Autodesk Inventor part; units mm, degrees
(part 2 of 2)
  spline S24 degree 3 poles (-22.161672, 44.941631) (-22.171925, 44.941805) (-22.192142, 44.942146) (-22.222099, 44.94568) (-22.251175, 44.951361) (-22.279514, 44.959316) (-22.307263, 44.969053) (-22.334041, 44.981738) (-22.360148, 44.996348) (-22.385514, 45.012986) (-22.409661, 45.032049) (-22.432726, 45.053133) (-22.45413, 45.076764) (-22.474051, 45.10257) (-22.492984, 45.130314) (-22.5104, 45.160373) (-22.526509, 45.192628) (-22.541234, 45.227289) (-22.554289, 45.264861) (-22.565821, 45.305774) (-22.574927, 45.350388) (-22.58272, 45.398346) (-22.589006, 45.449854) (-22.593298, 45.504939) (-22.595951, 45.563567) (-22.596186, 45.603781) (-22.596308, 45.624444) knots 0 0 0 0 0.03378715 0.06662166 0.09928488 0.13136117 0.16358519 0.19610393 0.22890225 0.26215806 0.29599122 0.33021785 0.36505983 0.40095074 0.43762038 0.47570753 0.51538069 0.55641354 0.59976483 0.64642416 0.69643144 0.74978152 0.80657331 0.86743553 0.93188675 1 1 1 1
  spline S25 degree 3 poles (-22.596308, 45.624444) (-22.596186, 45.64528) (-22.595949, 45.685755) (-22.593316, 45.744732) (-22.588943, 45.80006) (-22.582949, 45.851742) (-22.575655, 45.89979) (-22.565917, 45.944077) (-22.554844, 45.984808) (-22.54201, 46.022115) (-22.527529, 46.056501) (-22.511768, 46.088602) (-22.494101, 46.118369) (-22.475538, 46.146277) (-22.455328, 46.17187) (-22.434045, 46.195509) (-22.41086, 46.216647) (-22.38656, 46.235904) (-22.360926, 46.252786) (-22.334687, 46.267655) (-22.307663, 46.280358) (-22.279782, 46.290346) (-22.251292, 46.298595) (-22.222095, 46.304237) (-22.192143, 46.307787) (-22.171925, 46.308126) (-22.161672, 46.308298) knots 0 0 0 0 0.06859462 0.13324604 0.19431259 0.25127922 0.30451344 0.35423491 0.40048059 0.44341075 0.48401487 0.5232523 0.56104237 0.59790024 0.63351849 0.66831435 0.70249567 0.73668535 0.77029317 0.80343726 0.83591295 0.86846025 0.90084654 0.93346652 0.96625758 1 1 1 1
  spline S26 degree 3 poles (-22.161672, 46.308298) (-22.151333, 46.308117) (-22.130772, 46.307757) (-22.100375, 46.304293) (-22.070679, 46.298547) (-22.041812, 46.290405) (-22.013537, 46.280304) (-21.986075, 46.267643) (-21.959255, 46.252905) (-21.933504, 46.235587) (-21.908539, 46.21628) (-21.884972, 46.194454) (-21.862803, 46.170329) (-21.841752, 46.144165) (-21.822417, 46.115459) (-21.804004, 46.084711) (-21.787523, 46.051382) (-21.77165, 46.01603) (-21.757949, 45.977675) (-21.745593, 45.936533) (-21.73561, 45.89212) (-21.727294, 45.844668) (-21.720851, 45.794002) (-21.716159, 45.740232) (-21.713681, 45.683321) (-21.713214, 45.644411) (-21.712974, 45.624444) knots 0 0 0 0 0.03378812 0.06719393 0.09986241 0.13256661 0.16515117 0.19791319 0.231319 0.26508328 0.29925531 0.33439857 0.36994282 0.40628356 0.44406382 0.48299771 0.52335445 0.56553659 0.60961292 0.65639081 0.70588549 0.7583245 0.81383178 0.87279456 0.93472223 1 1 1 1
  line L64 (-27.862974, 45.624965) -> (-27.729641, 46.274965)
  line L65 (-27.729641, 46.274965) -> (-27.196308, 46.274965)
  line L66 (-27.196308, 46.274965) -> (-27.196308, 46.141631)
  line L67 (-27.196308, 46.141631) -> (-27.638495, 46.141631)
  line L68 (-27.638495, 46.141631) -> (-27.708547, 45.799704)
  spline S27 degree 3 poles (-27.708547, 45.799704) (-27.694784, 45.803504) (-27.668119, 45.810866) (-27.628762, 45.819039) (-27.591399, 45.823966) (-27.567154, 45.824639) (-27.555422, 45.824965) knots 0 0 0 0 0.27506837 0.53290146 0.77397346 1 1 1 1
  spline S28 degree 3 poles (-27.555422, 45.824965) (-27.540905, 45.824651) (-27.512362, 45.824033) (-27.470599, 45.8181) (-27.430732, 45.808763) (-27.392846, 45.795718) (-27.356869, 45.779037) (-27.323133, 45.7582) (-27.291131, 45.733859) (-27.261438, 45.705874) (-27.234501, 45.675074) (-27.210816, 45.641959) (-27.190699, 45.606848) (-27.174519, 45.569408) (-27.161599, 45.530052) (-27.153, 45.488365) (-27.147274, 45.444742) (-27.146634, 45.414914) (-27.146308, 45.399704) knots 0 0 0 0 0.06580765 0.12939427 0.19089406 0.25128107 0.31081496 0.37037099 0.43076826 0.49288125 0.55510395 0.61606705 0.67725603 0.73825981 0.80076213 0.86477758 0.93104529 1 1 1 1
  spline S29 degree 3 poles (-27.146308, 45.399704) (-27.146555, 45.38911) (-27.147045, 45.368066) (-27.149541, 45.336812) (-27.154346, 45.30622) (-27.160796, 45.276286) (-27.169169, 45.247066) (-27.179305, 45.218476) (-27.191709, 45.190695) (-27.205315, 45.16346) (-27.220636, 45.137387) (-27.237639, 45.113003) (-27.255603, 45.089943) (-27.274933, 45.068454) (-27.295808, 45.048678) (-27.317974, 45.030498) (-27.341257, 45.013604) (-27.366014, 44.998685) (-27.391696, 44.984956) (-27.418672, 44.973693) (-27.446329, 44.963623) (-27.475064, 44.955597) (-27.504813, 44.949307) (-27.535625, 44.945036) (-27.567338, 44.941925) (-27.588834, 44.94173) (-27.599693, 44.941631) knots 0 0 0 0 0.04401447 0.08743412 0.1301184 0.17255369 0.21455476 0.25629809 0.29843823 0.340849 0.38271519 0.42392405 0.46424624 0.50407367 0.54386191 0.58356672 0.62309432 0.66322906 0.70355126 0.74393789 0.78454125 0.82575011 0.86775736 0.91074516 0.95491445 1 1 1 1
  spline S30 degree 3 poles (-27.599693, 44.941631) (-27.612646, 44.941888) (-27.63813, 44.942393) (-27.675467, 44.947674) (-27.711389, 44.955238) (-27.745609, 44.966617) (-27.778432, 44.980875) (-27.809418, 44.998895) (-27.839357, 45.019316) (-27.867033, 45.043415) (-27.89272, 45.069755) (-27.915714, 45.098339) (-27.936192, 45.128696) (-27.953826, 45.160972) (-27.968869, 45.195084) (-27.980686, 45.231158) (-27.990223, 45.269006) (-27.994258, 45.295063) (-27.996308, 45.308298) knots 0 0 0 0 0.06542114 0.12870837 0.19023614 0.2507244 0.31063718 0.37076641 0.43161474 0.49352297 0.55588346 0.61734237 0.67866804 0.74071136 0.80298536 0.86680258 0.93234717 1 1 1 1
  line L69 (-27.996308, 45.308298) -> (-27.879641, 45.308298)
  spline S31 degree 3 poles (-27.879641, 45.308298) (-27.87677, 45.295901) (-27.871253, 45.272073) (-27.859142, 45.238596) (-27.844335, 45.208763) (-27.826728, 45.18218) (-27.805723, 45.159) (-27.781755, 45.138342) (-27.754883, 45.119706) (-27.725023, 45.104171) (-27.693521, 45.090923) (-27.66055, 45.082101) (-27.627008, 45.075898) (-27.604322, 45.075277) (-27.592922, 45.074965) knots 0 0 0 0 0.09468725 0.18199416 0.26437695 0.34217986 0.41861761 0.49650908 0.57736909 0.66151059 0.74673255 0.83125798 0.91520562 1 1 1 1
  spline S32 degree 3 poles (-27.592922, 45.074965) (-27.581795, 45.07527) (-27.559885, 45.07587) (-27.527641, 45.08049) (-27.49651, 45.087606) (-27.4668, 45.098255) (-27.437992, 45.111197) (-27.410813, 45.127805) (-27.384478, 45.146919) (-27.359804, 45.168817) (-27.337207, 45.192949) (-27.31724, 45.218755) (-27.300609, 45.246284) (-27.286593, 45.27506) (-27.275951, 45.305397) (-27.268358, 45.337155) (-27.2639, 45.370411) (-27.263287, 45.393094) (-27.262974, 45.404652) knots 0 0 0 0 0.0642073 0.12642469 0.18768028 0.24821642 0.30830506 0.36966099 0.43169855 0.49594689 0.55975802 0.62229541 0.68391064 0.74509241 0.80674023 0.86908662 0.93329 1 1 1 1
  spline S33 degree 3 poles (-27.262974, 45.404652) (-27.263219, 45.41508) (-27.263698, 45.435492) (-27.267609, 45.465355) (-27.274412, 45.49361) (-27.283856, 45.520396) (-27.295845, 45.545736) (-27.310497, 45.569657) (-27.328085, 45.591844) (-27.348176, 45.612307) (-27.370186, 45.631192) (-27.394494, 45.647291) (-27.420591, 45.660835) (-27.448162, 45.672523) (-27.477863, 45.680918) (-27.509106, 45.68722) (-27.542229, 45.690866) (-27.564875, 45.691371) (-27.576516, 45.691631) knots 0 0 0 0 0.06535138 0.12791603 0.18836021 0.24721608 0.30563013 0.36376984 0.42266091 0.48268729 0.54330022 0.60411796 0.66496489 0.72741349 0.79146763 0.85805544 0.92703681 1 1 1 1
  spline S34 degree 3 poles (-27.576516, 45.691631) (-27.586592, 45.691416) (-27.607398, 45.690971) (-27.639312, 45.687692) (-27.672849, 45.682403) (-27.70788, 45.675128) (-27.74451, 45.665608) (-27.782663, 45.6542) (-27.822418, 45.64056) (-27.849204, 45.63026) (-27.862974, 45.624965) knots 0 0 0 0 0.10220304 0.21102334 0.32509966 0.4465021 0.57378772 0.70890071 0.85035787 1 1 1 1
  line L70 (0, 0) -> (-7.5, 0)
  circle A17 centre (0, 0) radius 7.5
  line L71 (-11.162974, -50.524965) -> (-11.675559, -50.524965)
  line L72 (-11.675559, -50.524965) -> (-11.767254, -49.090957)
  arc A18 (-11.767254, -49.090957) -> (-15.958694, -49.090957) centre (-13.862974, -49.224965) ccw
  line L73 (-15.958694, -49.090957) -> (-16.05039, -50.524965)
  line L74 (-16.05039, -50.524965) -> (-20.33871, -50.524965)
  arc A19 (-20.409421, -50.495675) -> (-20.33871, -50.524965) centre (-20.33871, -50.424965) ccw
  line L75 (-20.409421, -50.495675) -> (-20.733685, -50.171411)
  arc A20 (-20.733685, -50.171411) -> (-21.087238, -50.024965) centre (-21.087238, -50.524965) ccw
  line L76 (-21.087238, -50.024965) -> (-30.762974, -50.024965)
  arc A21 (-30.862974, -49.924965) -> (-30.762974, -50.024965) centre (-30.762974, -49.924965) ccw
  line L77 (-30.862974, -49.924965) -> (-30.862974, -40.774965)
  arc A22 (-30.762974, -40.674965) -> (-30.862974, -40.774965) centre (-30.762974, -40.774965) ccw
  line L78 (-30.762974, -40.674965) -> (-27.837238, -40.674965)
  arc A23 (-27.837238, -40.674965) -> (-27.483685, -40.528518) centre (-27.837238, -40.174965) ccw
  line L79 (-27.483685, -40.528518) -> (-27.159421, -40.204254)
  arc A24 (-27.08871, -40.174965) -> (-27.159421, -40.204254) centre (-27.08871, -40.274965) ccw
  line L80 (-27.08871, -40.174965) -> (-24.337238, -40.174965)
  arc A25 (-24.266528, -40.204254) -> (-24.337238, -40.174965) centre (-24.337238, -40.274965) ccw
  line L81 (-24.266528, -40.204254) -> (-23.942264, -40.528518)
  arc A26 (-23.942264, -40.528518) -> (-23.58871, -40.674965) centre (-23.58871, -40.174965) ccw
  line L82 (-23.58871, -40.674965) -> (-18.337238, -40.674965)
  arc A27 (-18.337238, -40.674965) -> (-17.983685, -40.528518) centre (-18.337238, -40.174965) ccw
  line L83 (-17.983685, -40.528518) -> (-17.659421, -40.204254)
  arc A28 (-17.58871, -40.174965) -> (-17.659421, -40.204254) centre (-17.58871, -40.274965) ccw
  line L84 (-17.58871, -40.174965) -> (-14.837238, -40.174965)
  arc A29 (-14.766528, -40.204254) -> (-14.837238, -40.174965) centre (-14.837238, -40.274965) ccw
  line L85 (-14.766528, -40.204254) -> (-14.442264, -40.528518)
  arc A30 (-14.442264, -40.528518) -> (-14.08871, -40.674965) centre (-14.08871, -40.174965) ccw
  line L86 (-14.08871, -40.674965) -> (-11.162974, -40.674965)
  arc A31 (-11.062974, -40.774965) -> (-11.162974, -40.674965) centre (-11.162974, -40.774965) ccw
  line L87 (-11.062974, -40.774965) -> (-11.062974, -50.424965)
  arc A32 (-11.162974, -50.524965) -> (-11.062974, -50.424965) centre (-11.162974, -50.424965) ccw
  circle A33 centre (-16.212974, -42.724965) radius 1.25
  circle A34 centre (-25.712974, -42.724965) radius 1.25
  line L88 (-26.886308, -44.974965) -> (-26.269641, -46.274965)
  line L89 (-26.269641, -46.274965) -> (-26.252974, -46.274965)
  line L90 (-26.252974, -46.274965) -> (-25.652974, -44.974965)
  line L91 (-25.652974, -44.974965) -> (-25.779797, -44.974965)
  line L92 (-25.779797, -44.974965) -> (-25.971985, -45.391631)
  line L93 (-25.971985, -45.391631) -> (-26.561308, -45.391631)
  line L94 (-26.561308, -45.391631) -> (-26.758964, -44.974965)
  line L95 (-26.758964, -44.974965) -> (-26.886308, -44.974965)
  spline S35 degree 3 poles (-24.066308, -45.911423) (-24.066544, -45.920293) (-24.067009, -45.937775) (-24.071116, -45.963406) (-24.077323, -45.98813) (-24.086217, -46.012023) (-24.097957, -46.034846) (-24.112247, -46.056625) (-24.128734, -46.077681) (-24.147808, -46.097424) (-24.168761, -46.115506) (-24.190896, -46.131523) (-24.214314, -46.144909) (-24.238918, -46.155882) (-24.264637, -46.16449) (-24.291523, -46.170455) (-24.319501, -46.1742) (-24.338605, -46.174707) (-24.348339, -46.174965) knots 0 0 0 0 0.0619654 0.12212191 0.1809885 0.23993322 0.29990583 0.35998885 0.42177574 0.48657583 0.5515348 0.61501754 0.67725862 0.73972996 0.8030501 0.86649513 0.93197347 1 1 1 1
  spline S36 degree 3 poles (-24.348339, -46.174965) (-24.358505, -46.174699) (-24.37847, -46.174178) (-24.407783, -46.170529) (-24.435746, -46.164235) (-24.46243, -46.155627) (-24.48788, -46.144685) (-24.511973, -46.131056) (-24.534653, -46.114794) (-24.555965, -46.096356) (-24.5756, -46.075828) (-24.592851, -46.052944) (-24.607926, -46.028123) (-24.621078, -46.00143) (-24.631758, -45.972625) (-24.63992, -45.941808) (-24.646378, -45.909114) (-24.648535, -45.886537) (-24.649641, -45.874965) knots 0 0 0 0 0.06443867 0.12654691 0.18688715 0.24587754 0.30404088 0.36219122 0.42097593 0.48066028 0.54060027 0.6006891 0.66193579 0.72444251 0.78903839 0.85631376 0.92635203 1 1 1 1
  line L96 (-24.649641, -45.874965) -> (-24.766308, -45.874965)
  spline S37 degree 3 poles (-24.766308, -45.874965) (-24.765547, -45.890443) (-24.764054, -45.92084) (-24.757061, -45.965161) (-24.747054, -46.007524) (-24.732906, -46.04759) (-24.715335, -46.085713) (-24.694264, -46.121741) (-24.669306, -46.155538) (-24.641001, -46.18679) (-24.610258, -46.215459) (-24.577087, -46.240217) (-24.54223, -46.261135) (-24.505793, -46.278622) (-24.467365, -46.291749) (-24.427294, -46.301488) (-24.385405, -46.307348) (-24.356865, -46.307978) (-24.342349, -46.308298) knots 0 0 0 0 0.06879079 0.13510329 0.19897867 0.2619043 0.32349497 0.38519538 0.44696924 0.50976478 0.57225057 0.63340518 0.69325116 0.75258316 0.81257927 0.87327508 0.93554994 1 1 1 1
  spline S38 degree 3 poles (-24.342349, -46.308298) (-24.328095, -46.307964) (-24.300085, -46.307309) (-24.259204, -46.301677) (-24.220287, -46.292858) (-24.183409, -46.280483) (-24.148864, -46.263849) (-24.116392, -46.243867) (-24.085608, -46.220757) (-24.057897, -46.193548) (-24.032451, -46.164502) (-24.010499, -46.133492) (-23.9917, -46.101464) (-23.97603, -46.068173) (-23.964495, -46.033307) (-23.955737, -45.997372) (-23.950787, -45.959998) (-23.950027, -45.934701) (-23.949641, -45.92184) knots 0 0 0 0 0.06947546 0.1365168 0.20078882 0.26382967 0.32573502 0.38729069 0.44950922 0.51296782 0.57627522 0.6375801 0.69790261 0.75717209 0.81659853 0.87665317 0.93728964 1 1 1 1
  spline S39 degree 3 poles (-23.949641, -45.92184) (-23.95027, -45.903733) (-23.951517, -45.867838) (-23.962182, -45.81509) (-23.978839, -45.763984) (-23.998895, -45.722853) (-24.019128, -45.689709) (-24.037361, -45.662421) (-24.058705, -45.633039) (-24.083471, -45.601661) (-24.111147, -45.568043) (-24.141984, -45.532204) (-24.176201, -45.494514) (-24.200217, -45.468772) (-24.212662, -45.455434) knots 0 0 0 0 0.0987022 0.19567231 0.29242243 0.39134254 0.44446244 0.50422878 0.57035234 0.64254575 0.72228751 0.80792112 0.90046954 1 1 1 1
  line L97 (-24.212662, -45.455434) -> (-24.537922, -45.108298)
  line L98 (-24.537922, -45.108298) -> (-23.932974, -45.108298)
  line L99 (-23.932974, -45.108298) -> (-23.932974, -44.974965)
  line L100 (-23.932974, -44.974965) -> (-24.816308, -44.974965)
  line L101 (-24.816308, -44.974965) -> (-24.312141, -45.512986)
  spline S40 degree 3 poles (-24.312141, -45.512986) (-24.299866, -45.525799) (-24.276288, -45.550412) (-24.242941, -45.586345) (-24.212989, -45.61968) (-24.18624, -45.650355) (-24.163273, -45.678818) (-24.142892, -45.704148) (-24.126562, -45.727457) (-24.108839, -45.754475) (-24.091674, -45.787462) (-24.076923, -45.827775) (-24.067929, -45.869273) (-24.06685, -45.897317) (-24.066308, -45.911423) knots 0 0 0 0 0.11080264 0.2128292 0.30610131 0.39064732 0.46692447 0.53448104 0.59358694 0.644557 0.73620045 0.82502403 0.91198558 1 1 1 1
  line L102 (-23.556308, -45.624965) -> (-23.422974, -46.274965)
  line L103 (-23.422974, -46.274965) -> (-22.889641, -46.274965)
  line L104 (-22.889641, -46.274965) -> (-22.889641, -46.141631)
  line L105 (-22.889641, -46.141631) -> (-23.331828, -46.141631)
  line L106 (-23.331828, -46.141631) -> (-23.401881, -45.799704)
  spline S41 degree 3 poles (-23.401881, -45.799704) (-23.388117, -45.803504) (-23.361452, -45.810866) (-23.322096, -45.819039) (-23.284733, -45.823966) (-23.260488, -45.824639) (-23.248756, -45.824965) knots 0 0 0 0 0.27506837 0.53290146 0.77397346 1 1 1 1
  spline S42 degree 3 poles (-23.248756, -45.824965) (-23.234239, -45.824651) (-23.205695, -45.824033) (-23.163932, -45.8181) (-23.124065, -45.808763) (-23.086179, -45.795718) (-23.050202, -45.779037) (-23.016466, -45.7582) (-22.984465, -45.733859) (-22.954772, -45.705874) (-22.927834, -45.675074) (-22.90415, -45.641959) (-22.884032, -45.606848) (-22.867852, -45.569408) (-22.854932, -45.530052) (-22.846333, -45.488365) (-22.840607, -45.444742) (-22.839967, -45.414914) (-22.839641, -45.399704) knots 0 0 0 0 0.06580765 0.12939427 0.19089406 0.25128107 0.31081496 0.37037099 0.43076826 0.49288125 0.55510395 0.61606705 0.67725603 0.73825981 0.80076213 0.86477758 0.93104529 1 1 1 1
  spline S43 degree 3 poles (-22.839641, -45.399704) (-22.839888, -45.38911) (-22.840379, -45.368066) (-22.842874, -45.336812) (-22.847679, -45.30622) (-22.85413, -45.276286) (-22.862503, -45.247066) (-22.872639, -45.218476) (-22.885043, -45.190695) (-22.898649, -45.16346) (-22.913969, -45.137387) (-22.930972, -45.113003) (-22.948937, -45.089943) (-22.968266, -45.068454) (-22.989141, -45.048678) (-23.011308, -45.030498) (-23.03459, -45.013604) (-23.059348, -44.998685) (-23.085029, -44.984956) (-23.112005, -44.973693) (-23.139662, -44.963623) (-23.168398, -44.955597) (-23.198147, -44.949307) (-23.228959, -44.945036) (-23.260671, -44.941925) (-23.282168, -44.94173) (-23.293026, -44.941631) knots 0 0 0 0 0.04401447 0.08743412 0.1301184 0.17255369 0.21455476 0.25629809 0.29843823 0.340849 0.38271519 0.42392405 0.46424624 0.50407367 0.54386191 0.58356672 0.62309432 0.66322906 0.70355126 0.74393789 0.78454125 0.82575011 0.86775736 0.91074516 0.95491445 1 1 1 1
  spline S44 degree 3 poles (-23.293026, -44.941631) (-23.30598, -44.941888) (-23.331464, -44.942393) (-23.3688, -44.947674) (-23.404722, -44.955238) (-23.438942, -44.966617) (-23.471766, -44.980875) (-23.502751, -44.998895) (-23.532691, -45.019316) (-23.560367, -45.043415) (-23.586053, -45.069755) (-23.609047, -45.098339) (-23.629525, -45.128696) (-23.64716, -45.160972) (-23.662202, -45.195084) (-23.674019, -45.231158) (-23.683557, -45.269006) (-23.687592, -45.295063) (-23.689641, -45.308298) knots 0 0 0 0 0.06542114 0.12870837 0.19023614 0.2507244 0.31063718 0.37076641 0.43161474 0.49352297 0.55588346 0.61734237 0.67866804 0.74071136 0.80298536 0.86680258 0.93234717 1 1 1 1
  line L107 (-23.689641, -45.308298) -> (-23.572974, -45.308298)
  spline S45 degree 3 poles (-23.572974, -45.308298) (-23.570104, -45.295901) (-23.564586, -45.272073) (-23.552475, -45.238596) (-23.537668, -45.208763) (-23.520061, -45.18218) (-23.499057, -45.159) (-23.475088, -45.138342) (-23.448216, -45.119706) (-23.418356, -45.104171) (-23.386854, -45.090923) (-23.353883, -45.082101) (-23.320342, -45.075898) (-23.297656, -45.075277) (-23.286256, -45.074965) knots 0 0 0 0 0.09468725 0.18199416 0.26437695 0.34217986 0.41861761 0.49650908 0.57736909 0.66151059 0.74673255 0.83125798 0.91520562 1 1 1 1
  spline S46 degree 3 poles (-23.286256, -45.074965) (-23.275128, -45.07527) (-23.253218, -45.07587) (-23.220974, -45.08049) (-23.189843, -45.087606) (-23.160134, -45.098255) (-23.131325, -45.111197) (-23.104146, -45.127805) (-23.077811, -45.146919) (-23.053138, -45.168817) (-23.03054, -45.192949) (-23.010574, -45.218755) (-22.993942, -45.246284) (-22.979927, -45.27506) (-22.969284, -45.305397) (-22.961692, -45.337155) (-22.957233, -45.370411) (-22.95662, -45.393094) (-22.956308, -45.404652) knots 0 0 0 0 0.0642073 0.12642469 0.18768028 0.24821642 0.30830506 0.36966099 0.43169855 0.49594689 0.55975802 0.62229541 0.68391064 0.74509241 0.80674023 0.86908662 0.93329 1 1 1 1
  spline S47 degree 3 poles (-22.956308, -45.404652) (-22.956552, -45.41508) (-22.957031, -45.435492) (-22.960942, -45.465355) (-22.967746, -45.49361) (-22.977189, -45.520396) (-22.989178, -45.545736) (-23.00383, -45.569657) (-23.021418, -45.591844) (-23.04151, -45.612307) (-23.06352, -45.631192) (-23.087827, -45.647291) (-23.113924, -45.660835) (-23.141495, -45.672523) (-23.171196, -45.680918) (-23.202439, -45.68722) (-23.235562, -45.690866) (-23.258209, -45.691371) (-23.269849, -45.691631) knots 0 0 0 0 0.06535138 0.12791603 0.18836021 0.24721608 0.30563013 0.36376984 0.42266091 0.48268729 0.54330022 0.60411796 0.66496489 0.72741349 0.79146763 0.85805544 0.92703681 1 1 1 1
  spline S48 degree 3 poles (-23.269849, -45.691631) (-23.279926, -45.691416) (-23.300731, -45.690971) (-23.332645, -45.687692) (-23.366182, -45.682403) (-23.401213, -45.675128) (-23.437844, -45.665608) (-23.475996, -45.6542) (-23.515751, -45.64056) (-23.542538, -45.63026) (-23.556308, -45.624965) knots 0 0 0 0 0.10220304 0.21102334 0.32509966 0.4465021 0.57378772 0.70890071 0.85035787 1 1 1 1
  line L108 (-20.109641, -44.974965) -> (-19.492974, -46.274965)
  line L109 (-19.492974, -46.274965) -> (-19.476308, -46.274965)
  line L110 (-19.476308, -46.274965) -> (-18.876308, -44.974965)
  line L111 (-18.876308, -44.974965) -> (-19.003131, -44.974965)
  line L112 (-19.003131, -44.974965) -> (-19.195318, -45.391631)
  line L113 (-19.195318, -45.391631) -> (-19.784641, -45.391631)
  line L114 (-19.784641, -45.391631) -> (-19.982297, -44.974965)
  line L115 (-19.982297, -44.974965) -> (-20.109641, -44.974965)
  spline S49 degree 3 poles (-18.599641, -45.632517) (-18.599063, -45.6559) (-18.597927, -45.701906) (-18.588271, -45.769422) (-18.572739, -45.834107) (-18.550677, -45.895839) (-18.522706, -45.954945) (-18.488154, -46.010972) (-18.44742, -46.064278) (-18.400825, -46.114055) (-18.349729, -46.159569) (-18.29501, -46.199612) (-18.236777, -46.232935) (-18.17567, -46.260791) (-18.111233, -46.282202) (-18.043602, -46.29719) (-17.972905, -46.306519) (-17.92467, -46.307699) (-17.900162, -46.308298) knots 0 0 0 0 0.06455785 0.12701353 0.18795481 0.24801391 0.30774768 0.36823451 0.42946984 0.49274344 0.55625777 0.61821679 0.67965548 0.74124555 0.80341526 0.86681546 0.93232831 1 1 1 1
  spline S50 degree 3 poles (-17.900162, -46.308298) (-17.885225, -46.308119) (-17.855659, -46.307765) (-17.811922, -46.304308) (-17.769341, -46.298546) (-17.727885, -46.290703) (-17.687354, -46.280969) (-17.648057, -46.268288) (-17.609763, -46.253789) (-17.572714, -46.23709) (-17.537088, -46.218345) (-17.502896, -46.197762) (-17.470409, -46.175366) (-17.439399, -46.151349) (-17.410384, -46.125201) (-17.382541, -46.097641) (-17.356816, -46.067877) (-17.340936, -46.046927) (-17.332974, -46.036423) knots 0 0 0 0 0.06854754 0.13568295 0.20121499 0.26568223 0.32926683 0.39239543 0.45506976 0.51712685 0.57879004 0.63973986 0.7001915 0.75980624 0.81962832 0.87935479 0.93951161 1 1 1 1
  line L116 (-17.332974, -46.036423) -> (-17.435058, -45.958298)
  spline S51 degree 3 poles (-17.435058, -45.958298) (-17.44234, -45.966977) (-17.456806, -45.984217) (-17.480079, -46.008427) (-17.504334, -46.031108) (-17.529561, -46.05237) (-17.556215, -46.071467) (-17.583649, -46.089397) (-17.612322, -46.105467) (-17.651973, -46.124954) (-17.703842, -46.145288) (-17.769137, -46.162338) (-17.837299, -46.173191) (-17.883801, -46.174367) (-17.907453, -46.174965) knots 0 0 0 0 0.06316326 0.12547494 0.18712122 0.24829435 0.30929486 0.36985007 0.43097338 0.49245599 0.61614797 0.7408437 0.86818265 1 1 1 1
  spline S52 degree 3 poles (-17.907453, -46.174965) (-17.920484, -46.174815) (-17.946425, -46.174516) (-17.984923, -46.170575) (-18.022702, -46.165037) (-18.059738, -46.156819) (-18.095983, -46.146429) (-18.131675, -46.134014) (-18.166296, -46.118654) (-18.200325, -46.101676) (-18.232929, -46.0825) (-18.263778, -46.061584) (-18.29276, -46.039161) (-18.319897, -46.015148) (-18.345219, -45.989652) (-18.36854, -45.962403) (-18.38978, -45.933486) (-18.40936, -45.903284) (-18.426897, -45.871884) (-18.441579, -45.839171) (-18.454581, -45.805704) (-18.464869, -45.771105) (-18.473013, -45.735617) (-18.478632, -45.699146) (-18.482527, -45.661768) (-18.482824, -45.636433) (-18.482974, -45.623663) knots 0 0 0 0 0.04395491 0.08750187 0.13046263 0.17275202 0.21540307 0.25764983 0.30015275 0.34312149 0.38592516 0.42768573 0.46881795 0.5094918 0.54988303 0.58998002 0.63040523 0.67086863 0.71138394 0.75162726 0.79177558 0.83245892 0.87331905 0.91454296 0.95692356 1 1 1 1
  spline S53 degree 3 poles (-18.482974, -45.623663) (-18.482506, -45.604448) (-18.481585, -45.566723) (-18.473396, -45.511465) (-18.460951, -45.458529) (-18.4423, -45.408245) (-18.419301, -45.359994) (-18.39024, -45.314591) (-18.356583, -45.27135) (-18.317852, -45.231294) (-18.275359, -45.194703) (-18.229767, -45.162482) (-18.18119, -45.135622) (-18.130164, -45.113271) (-18.076297, -45.09609) (-18.019686, -45.083995) (-17.960454, -45.076105) (-17.919979, -45.075349) (-17.899381, -45.074965) knots 0 0 0 0 0.06432322 0.1262901 0.18672647 0.24614643 0.30557564 0.36542939 0.42632631 0.48883991 0.55172497 0.6139186 0.67548377 0.7373339 0.80022904 0.8645023 0.93104074 1 1 1 1
  spline S54 degree 3 poles (-17.899381, -45.074965) (-17.876685, -45.075592) (-17.832015, -45.076827) (-17.766507, -45.087286) (-17.703797, -45.104244) (-17.643881, -45.127978) (-17.586928, -45.158831) (-17.532849, -45.196233) (-17.481599, -45.24054) (-17.450781, -45.274371) (-17.435058, -45.291631) knots 0 0 0 0 0.12851519 0.25294864 0.37475473 0.49593975 0.61718064 0.74090947 0.86781115 1 1 1 1
  line L117 (-17.435058, -45.291631) -> (-17.332974, -45.214288)
  spline S55 degree 3 poles (-17.332974, -45.214288) (-17.34119, -45.203688) (-17.357581, -45.182538) (-17.384122, -45.152723) (-17.412083, -45.124679) (-17.441669, -45.098631) (-17.472541, -45.07406) (-17.505254, -45.051662) (-17.539377, -45.031125) (-17.574794, -45.012321) (-17.611468, -44.995638) (-17.649356, -44.981355) (-17.688293, -44.969051) (-17.728281, -44.958929) (-17.769404, -44.951028) (-17.811513, -44.945747) (-17.854699, -44.942128) (-17.883835, -44.941799) (-17.898599, -44.941631) knots 0 0 0 0 0.06167424 0.12305306 0.183475 0.2437265 0.30427892 0.36486292 0.4259462 0.48739123 0.54922038 0.61114359 0.67352853 0.73696146 0.80078528 0.8660126 0.93210075 1 1 1 1
  spline S56 degree 3 poles (-17.898599, -44.941631) (-17.912581, -44.941729) (-17.940229, -44.941921) (-17.981048, -44.945038) (-18.020787, -44.949291) (-18.059332, -44.955694) (-18.096893, -44.963251) (-18.13313, -44.97338) (-18.168399, -44.984727) (-18.202559, -44.998063) (-18.235638, -45.013112) (-18.26753, -45.03012) (-18.298221, -45.048945) (-18.328011, -45.069171) (-18.356462, -45.091449) (-18.383819, -45.115468) (-18.410236, -45.141147) (-18.42658, -45.159665) (-18.434797, -45.168975) knots 0 0 0 0 0.0696628 0.13774956 0.20391674 0.26877986 0.33241371 0.39475354 0.45618003 0.51699565 0.57739594 0.63719834 0.69699918 0.75675619 0.81655391 0.876948 0.93813179 1 1 1 1
  spline S57 degree 3 poles (-18.434797, -45.168975) (-18.447959, -45.185148) (-18.474124, -45.217297) (-18.507599, -45.269403) (-18.536254, -45.323806) (-18.559422, -45.38079) (-18.577534, -45.440229) (-18.590081, -45.502152) (-18.598235, -45.566501) (-18.599167, -45.610269) (-18.599641, -45.632517) knots 0 0 0 0 0.12432851 0.24715602 0.36877975 0.49073386 0.61361377 0.73895758 0.86731058 1 1 1 1
  line L118 (-15.526977, -46.224965) -> (-15.739813, -46.224965)
  line L119 (-15.927345, -45.124965) -> (-15.526977, -46.224965)
  line L120 (-15.427345, -45.124965) -> (-15.927345, -45.124965)
  line L121 (-15.026977, -46.224965) -> (-15.427345, -45.124965)
  line L122 (-14.814142, -46.224965) -> (-15.026977, -46.224965)
  line L123 (-15.214509, -45.124965) -> (-14.814142, -46.224965)
  line L124 (-15.014509, -45.124965) -> (-15.214509, -45.124965)
  line L125 (-15.087303, -44.924965) -> (-15.014509, -45.124965)
  line L126 (-16.212974, -44.924965) -> (-15.087303, -44.924965)
  line L127 (-15.739813, -46.224965) -> (-16.212974, -44.924965)
  line L128 (-20.902974, -44.974965) -> (-20.919641, -44.974965)
  line L129 (-20.919641, -44.974965) -> (-21.469641, -46.274965)
  line L130 (-21.469641, -46.274965) -> (-21.344641, -46.274965)
  line L131 (-21.344641, -46.274965) -> (-20.911308, -45.250486)
  line L132 (-20.911308, -45.250486) -> (-20.477974, -46.274965)
  line L133 (-20.477974, -46.274965) -> (-20.352974, -46.274965)
  line L134 (-20.352974, -46.274965) -> (-20.902974, -44.974965)
  spline S58 degree 3 poles (-21.712974, -45.624444) (-21.713216, -45.604564) (-21.713688, -45.565828) (-21.716131, -45.509173) (-21.720945, -45.455688) (-21.726965, -45.405244) (-21.735304, -45.358052) (-21.745558, -45.313947) (-21.756942, -45.272739) (-21.770995, -45.234766) (-21.786376, -45.199498) (-21.803111, -45.166564) (-21.82104, -45.135674) (-21.840573, -45.107074) (-21.861393, -45.080562) (-21.883945, -45.056606) (-21.907594, -45.034628) (-21.932633, -45.015072) (-21.958786, -44.997955) (-21.985513, -44.982647) (-22.01329, -44.970303) (-22.041486, -44.959704) (-22.070505, -44.951607) (-22.100311, -44.946008) (-22.130752, -44.942082) (-22.15133, -44.941782) (-22.161672, -44.941631) knots 0 0 0 0 0.06506329 0.12677317 0.18551576 0.24076468 0.2929798 0.34225037 0.38891929 0.43277566 0.47462843 0.51477469 0.55360589 0.59142641 0.62802812 0.66380363 0.69898434 0.73359149 0.76762847 0.80120835 0.83426384 0.86698069 0.89971974 0.93270191 0.96617588 1 1 1 1
  spline S59 degree 3 poles (-22.161672, -44.941631) (-22.171925, -44.941805) (-22.192142, -44.942146) (-22.222099, -44.94568) (-22.251175, -44.951361) (-22.279514, -44.959316) (-22.307263, -44.969053) (-22.334041, -44.981738) (-22.360148, -44.996348) (-22.385514, -45.012986) (-22.409661, -45.032049) (-22.432726, -45.053133) (-22.45413, -45.076764) (-22.474051, -45.10257) (-22.492984, -45.130314) (-22.5104, -45.160373) (-22.526509, -45.192628) (-22.541234, -45.227289) (-22.554289, -45.264861) (-22.565821, -45.305774) (-22.574927, -45.350388) (-22.58272, -45.398346) (-22.589006, -45.449854) (-22.593298, -45.504939) (-22.595951, -45.563567) (-22.596186, -45.603781) (-22.596308, -45.624444) knots 0 0 0 0 0.03378715 0.06662166 0.09928488 0.13136117 0.16358519 0.19610393 0.22890225 0.26215806 0.29599122 0.33021785 0.36505983 0.40095074 0.43762038 0.47570753 0.51538069 0.55641354 0.59976483 0.64642416 0.69643144 0.74978152 0.80657331 0.86743553 0.93188675 1 1 1 1
  spline S60 degree 3 poles (-22.596308, -45.624444) (-22.596186, -45.64528) (-22.595949, -45.685755) (-22.593316, -45.744732) (-22.588943, -45.80006) (-22.582949, -45.851742) (-22.575655, -45.89979) (-22.565917, -45.944077) (-22.554844, -45.984808) (-22.54201, -46.022115) (-22.527529, -46.056501) (-22.511768, -46.088602) (-22.494101, -46.118369) (-22.475538, -46.146277) (-22.455328, -46.17187) (-22.434045, -46.195509) (-22.41086, -46.216647) (-22.38656, -46.235904) (-22.360926, -46.252786) (-22.334687, -46.267655) (-22.307663, -46.280358) (-22.279782, -46.290346) (-22.251292, -46.298595) (-22.222095, -46.304237) (-22.192143, -46.307787) (-22.171925, -46.308126) (-22.161672, -46.308298) knots 0 0 0 0 0.06859462 0.13324604 0.19431259 0.25127922 0.30451344 0.35423491 0.40048059 0.44341075 0.48401487 0.5232523 0.56104237 0.59790024 0.63351849 0.66831435 0.70249567 0.73668535 0.77029317 0.80343726 0.83591295 0.86846025 0.90084654 0.93346652 0.96625758 1 1 1 1
  spline S61 degree 3 poles (-22.161672, -46.308298) (-22.151333, -46.308117) (-22.130772, -46.307757) (-22.100375, -46.304293) (-22.070679, -46.298547) (-22.041812, -46.290405) (-22.013537, -46.280304) (-21.986075, -46.267643) (-21.959255, -46.252905) (-21.933504, -46.235587) (-21.908539, -46.21628) (-21.884972, -46.194454) (-21.862803, -46.170329) (-21.841752, -46.144165) (-21.822417, -46.115459) (-21.804004, -46.084711) (-21.787523, -46.051382) (-21.77165, -46.01603) (-21.757949, -45.977675) (-21.745593, -45.936533) (-21.73561, -45.89212) (-21.727294, -45.844668) (-21.720851, -45.794002) (-21.716159, -45.740232) (-21.713681, -45.683321) (-21.713214, -45.644411) (-21.712974, -45.624444) knots 0 0 0 0 0.03378812 0.06719393 0.09986241 0.13256661 0.16515117 0.19791319 0.231319 0.26508328 0.29925531 0.33439857 0.36994282 0.40628356 0.44406382 0.48299771 0.52335445 0.56553659 0.60961292 0.65639081 0.70588549 0.7583245 0.81383178 0.87279456 0.93472223 1 1 1 1
  line L135 (-27.862974, -45.624965) -> (-27.729641, -46.274965)
  line L136 (-27.729641, -46.274965) -> (-27.196308, -46.274965)
  line L137 (-27.196308, -46.274965) -> (-27.196308, -46.141631)
  line L138 (-27.196308, -46.141631) -> (-27.638495, -46.141631)
  line L139 (-27.638495, -46.141631) -> (-27.708547, -45.799704)
  spline S62 degree 3 poles (-27.708547, -45.799704) (-27.694784, -45.803504) (-27.668119, -45.810866) (-27.628762, -45.819039) (-27.591399, -45.823966) (-27.567154, -45.824639) (-27.555422, -45.824965) knots 0 0 0 0 0.27506837 0.53290146 0.77397346 1 1 1 1
  spline S63 degree 3 poles (-27.555422, -45.824965) (-27.540905, -45.824651) (-27.512362, -45.824033) (-27.470599, -45.8181) (-27.430732, -45.808763) (-27.392846, -45.795718) (-27.356869, -45.779037) (-27.323133, -45.7582) (-27.291131, -45.733859) (-27.261438, -45.705874) (-27.234501, -45.675074) (-27.210816, -45.641959) (-27.190699, -45.606848) (-27.174519, -45.569408) (-27.161599, -45.530052) (-27.153, -45.488365) (-27.147274, -45.444742) (-27.146634, -45.414914) (-27.146308, -45.399704) knots 0 0 0 0 0.06580765 0.12939427 0.19089406 0.25128107 0.31081496 0.37037099 0.43076826 0.49288125 0.55510395 0.61606705 0.67725603 0.73825981 0.80076213 0.86477758 0.93104529 1 1 1 1
  spline S64 degree 3 poles (-27.146308, -45.399704) (-27.146555, -45.38911) (-27.147045, -45.368066) (-27.149541, -45.336812) (-27.154346, -45.30622) (-27.160796, -45.276286) (-27.169169, -45.247066) (-27.179305, -45.218476) (-27.191709, -45.190695) (-27.205315, -45.16346) (-27.220636, -45.137387) (-27.237639, -45.113003) (-27.255603, -45.089943) (-27.274933, -45.068454) (-27.295808, -45.048678) (-27.317974, -45.030498) (-27.341257, -45.013604) (-27.366014, -44.998685) (-27.391696, -44.984956) (-27.418672, -44.973693) (-27.446329, -44.963623) (-27.475064, -44.955597) (-27.504813, -44.949307) (-27.535625, -44.945036) (-27.567338, -44.941925) (-27.588834, -44.94173) (-27.599693, -44.941631) knots 0 0 0 0 0.04401447 0.08743412 0.1301184 0.17255369 0.21455476 0.25629809 0.29843823 0.340849 0.38271519 0.42392405 0.46424624 0.50407367 0.54386191 0.58356672 0.62309432 0.66322906 0.70355126 0.74393789 0.78454125 0.82575011 0.86775736 0.91074516 0.95491445 1 1 1 1
  spline S65 degree 3 poles (-27.599693, -44.941631) (-27.612646, -44.941888) (-27.63813, -44.942393) (-27.675467, -44.947674) (-27.711389, -44.955238) (-27.745609, -44.966617) (-27.778432, -44.980875) (-27.809418, -44.998895) (-27.839357, -45.019316) (-27.867033, -45.043415) (-27.89272, -45.069755) (-27.915714, -45.098339) (-27.936192, -45.128696) (-27.953826, -45.160972) (-27.968869, -45.195084) (-27.980686, -45.231158) (-27.990223, -45.269006) (-27.994258, -45.295063) (-27.996308, -45.308298) knots 0 0 0 0 0.06542114 0.12870837 0.19023614 0.2507244 0.31063718 0.37076641 0.43161474 0.49352297 0.55588346 0.61734237 0.67866804 0.74071136 0.80298536 0.86680258 0.93234717 1 1 1 1
  line L140 (-27.996308, -45.308298) -> (-27.879641, -45.308298)
  spline S66 degree 3 poles (-27.879641, -45.308298) (-27.87677, -45.295901) (-27.871253, -45.272073) (-27.859142, -45.238596) (-27.844335, -45.208763) (-27.826728, -45.18218) (-27.805723, -45.159) (-27.781755, -45.138342) (-27.754883, -45.119706) (-27.725023, -45.104171) (-27.693521, -45.090923) (-27.66055, -45.082101) (-27.627008, -45.075898) (-27.604322, -45.075277) (-27.592922, -45.074965) knots 0 0 0 0 0.09468725 0.18199416 0.26437695 0.34217986 0.41861761 0.49650908 0.57736909 0.66151059 0.74673255 0.83125798 0.91520562 1 1 1 1
  spline S67 degree 3 poles (-27.592922, -45.074965) (-27.581795, -45.07527) (-27.559885, -45.07587) (-27.527641, -45.08049) (-27.49651, -45.087606) (-27.4668, -45.098255) (-27.437992, -45.111197) (-27.410813, -45.127805) (-27.384478, -45.146919) (-27.359804, -45.168817) (-27.337207, -45.192949) (-27.31724, -45.218755) (-27.300609, -45.246284) (-27.286593, -45.27506) (-27.275951, -45.305397) (-27.268358, -45.337155) (-27.2639, -45.370411) (-27.263287, -45.393094) (-27.262974, -45.404652) knots 0 0 0 0 0.0642073 0.12642469 0.18768028 0.24821642 0.30830506 0.36966099 0.43169855 0.49594689 0.55975802 0.62229541 0.68391064 0.74509241 0.80674023 0.86908662 0.93329 1 1 1 1
  spline S68 degree 3 poles (-27.262974, -45.404652) (-27.263219, -45.41508) (-27.263698, -45.435492) (-27.267609, -45.465355) (-27.274412, -45.49361) (-27.283856, -45.520396) (-27.295845, -45.545736) (-27.310497, -45.569657) (-27.328085, -45.591844) (-27.348176, -45.612307) (-27.370186, -45.631192) (-27.394494, -45.647291) (-27.420591, -45.660835) (-27.448162, -45.672523) (-27.477863, -45.680918) (-27.509106, -45.68722) (-27.542229, -45.690866) (-27.564875, -45.691371) (-27.576516, -45.691631) knots 0 0 0 0 0.06535138 0.12791603 0.18836021 0.24721608 0.30563013 0.36376984 0.42266091 0.48268729 0.54330022 0.60411796 0.66496489 0.72741349 0.79146763 0.85805544 0.92703681 1 1 1 1
  spline S69 degree 3 poles (-27.576516, -45.691631) (-27.586592, -45.691416) (-27.607398, -45.690971) (-27.639312, -45.687692) (-27.672849, -45.682403) (-27.70788, -45.675128) (-27.74451, -45.665608) (-27.782663, -45.6542) (-27.822418, -45.64056) (-27.849204, -45.63026) (-27.862974, -45.624965) knots 0 0 0 0 0.10220304 0.21102334 0.32509966 0.4465021 0.57378772 0.70890071 0.85035787 1 1 1 1
  dimension "d146" = 9.5
  constraints: 282 end point, 138 symmetric about line, 60 point on circle, 36 horizontal, 34 centre point, 1 horizontal alignment, 162 other
  measures "d146" distance of point (-16.213, 42.725) A16.centre
sketch "Эскиз31 outline for Выдавливание28" plane through (0, 0, 0) normal (0, -1, 0) x (1, 0, 0)
  circle A0 centre (-16.212974, 42.724965) radius 1.25
  circle A1 centre (-25.712974, 42.724965) radius 1.25
  circle A2 centre (-25.712974, -42.724965) radius 1.25
  circle A3 centre (-16.212974, -42.724965) radius 1.25
extrude "Выдавливание28" cut sketch "Эскиз31 outline for Выдавливание28" against normal blind 56.25
move faces "Перенос6" translate (3.25, 0, 0) faces at (-19, 4.521369, 33.275217) (-19, 4.521369, -26.724783)
sketch "Эскиз33" plane through (0, 10, 0) normal (0, 1, 0) x (1, 0, 0)
  circle A0 centre (-22.5, 13.5) radius 1.3 projected
  circle A1 centre (-22.5, 13.5) radius 2.5
  point P0 (0, 0)
  dimension "d150" = 5
  constraints: 1 centre point, 1 coincident
  measures "d150" diameter of A1
sketch "Эскиз33 outline for Выдавливание29" plane through (0, 10, 0) normal (0, 1, 0) x (1, 0, 0)
  circle A0 centre (-22.5, 13.5) radius 2.5
  circle A1 centre (-22.5, 13.5) radius 1.3
extrude "Выдавливание29" cut sketch "Эскиз33 outline for Выдавливание29" against normal up to surface (2 mm away)
